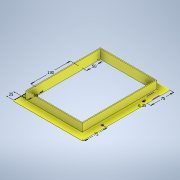
# Autodesk Inventor part: Tapa Superior
Saved by Autodesk Inventor 2022.6 (Build 266554000, 554)
## iProperties
Created: 2025-01-14
Part Number: Tapa Superior
Material: Genérico
Document SubType Name: Modeling
Designer: johan
Density: 1 g/cm^3
Appearance: Valor por defecto
Author: johan
Autodesk Inventor part; units mm, degrees
ref_plane "YZ Plane" through (0, 0, 0) normal (1, 0, 0) x (0, 1, 0)
ref_plane "XZ Plane" through (0, 0, 0) normal (0, 1, 0) x (-1, 0, 0)
ref_plane "XY Plane" through (0, 0, 0) normal (0, 0, 1) x (1, 0, 0)
sketch "Boceto1" plane through (0, 0, 0) normal (0, 1, 0) x (-1, 0, 0)
  line L0 (0, 0) -> (180, 0)
  line L1 (180, 0) -> (180, -240)
  line L2 (180, -240) -> (0, -240)
  line L3 (0, -240) -> (0, 0)
  line L4 (-3, -243) -> (183, -243)
  line L5 (183, -243) -> (183, 3)
  line L6 (183, 3) -> (-3, 3)
  line L7 (-3, 3) -> (-3, -243)
  line L8 (203, 23) -> (203, -263)
  line L9 (203, -263) -> (-23, -263)
  line L10 (-23, -263) -> (-23, 23)
  line L11 (-23, 23) -> (203, 23)
  dimension "d0" = 180
  dimension "d1" = 240
  dimension "d2" = 3
  dimension "d5" = 20
  constraints: 24 end point, 6 parallel, 3 perpendicular, 1 horizontal, 6 other
  measures "d0" distance of L1.end L2.end
  measures "d1" distance of L0.end L1.end
  measures "d2" distance between parallel lines of L2 L4
  measures "d5" distance between parallel lines of L5 L8
extrude "Extrusión2" add sketch "Boceto1" along normal blind 30 contours L7 L6 L5 L4
extrude "Extrusión3" add sketch "Boceto1" along normal blind 3 contours L8 L9 L10 L11
fillet "Empalme1" radius 2 4 edges at (3, 3, -120) (-90, 3, 3) (-90, 3, -243) (-183, 3, -120)
sketch "Boceto3" plane through (0, 3, 0) normal (0, 1, 0) x (1, 0, 0)
  line L0 (23, -23) -> (23, 263) projected
  line L1 (23, 263) -> (-203, 263) projected
  line L2 (-203, 263) -> (-203, -23) projected
  line L3 (-203, -23) -> (23, -23) projected
  line L4 (-185, -5) -> (5, -5) projected
  line L5 (-185, 245) -> (-185, -5) projected
  line L6 (5, 245) -> (-185, 245) projected
  line L7 (5, -5) -> (5, 245) projected
  line L8 (-203, 263) -> (-203, -23) projected
  line L9 (-203, -23) -> (-203, 2)
  line L10 (-185, 245) -> (-185, -5) projected
  line L11 (-203, 2) -> (-185, 2)
  line L12 (-185, 2) -> (-185, 52)
  line L13 (-185, 52) -> (-203, 52)
  line L14 (-203, 52) -> (-203, 2)
  line L15 (-183, 243) -> (-183, -3) projected
  line L16 (-203, 182) -> (-183, 182)
  line L17 (-183, 182) -> (-183, 232)
  line L18 (-183, 232) -> (-203, 232)
  line L19 (-203, 232) -> (-203, 182)
  line L20 (5, -5) -> (5, 245) projected
  line L21 (23, 207) -> (23, 232)
  line L22 (5, 232) -> (5, 207)
  circle A0 centre (14, 188) radius 3.175
  circle A1 centre (14, 52) radius 3.1767
  point P0 (0, 0)
  point P1 (-193, 182)
  point P2 (-185, 232)
  point P3 (-185, 182)
  dimension "d11" = 25
  dimension "d12" = 50
  dimension "d13" = 50
  dimension "d14" = 130
  dimension "d15" = 6.35
  dimension "d16" = 75
  dimension "d17" = 75
  constraints: 22 end point, 6 point on line, 5 parallel, 2 centre point, 2 horizontal, 2 perpendicular, 1 midpoint
  measures "d11" distance of L2.end L9.end
  measures "d12" distance of L12.end L11.end
  measures "d13" distance of L17.end L16.end
  measures "d14" distance from line of point (-193, 182) L13
  measures "d15" diameter of A0
  measures "d16" distance from line of L1 A0.centre
  measures "d17" distance from line of A1.centre L3
extrude "Extrusión5" cut sketch "Boceto3" against normal blind 3 contours A0 | A1
